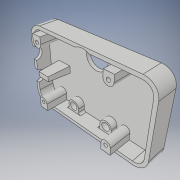
# Autodesk Inventor part: Case_Bottom
Saved by Autodesk Inventor 2019 (Build 230136000, 136)
## iProperties
Created: 2025-01-19
Part Number: Case_Bottom
Material: Générique
Document SubType Name: Modeling
Designer: Maxime
Density: 1 g/cm^3
Appearance: Par défaut
Author: Maxime
Autodesk Inventor part; units mm, degrees
ref_plane "XZ Plane" through (0, 0, 0) normal (0, 1, 0) x (-1, 0, 0)
ref_plane "XY Plane" through (0, 0, 0) normal (0, 0, 1) x (1, 0, 0)
sketch "Esquisse1" plane through (0, 0, 0) normal (0, 0, 1) x (1, 0, 0)
  line L0 (53.2, -33.2) -> (-53.2, -33.2)
  line L1 (-53.2, -33.2) -> (-53.2, 33.2)
  line L2 (-53.2, 33.2) -> (53.2, 33.2)
  line L3 (53.2, 33.2) -> (53.2, -33.2)
  line L4 (53.2, -33.2) -> (-53.2, 33.2) construction
  line L5 (-53.2, -33.2) -> (53.2, 33.2) construction
  point P0 (0, 0)
  dimension "d0" = 66.4
  dimension "d1" = 106.4
  constraints: 12 end point, 2 midpoint, 2 parallel, 1 horizontal, 1 perpendicular
  measures "d0" distance of L0.end L1.end
  measures "d1" distance between parallel lines of L3 L1
extrude "Extrusion1" add sketch "Esquisse1" along normal blind 15.95
shell "Coque1" thickness 3 removed faces 1 at (17.7333, 11.0667, 15.95)
ref_plane "PCBRestingPlane" through (-50.2, -30.2, 22.3) normal (0, 0, 1) x (1, 0, 0)
sketch "Esquisse2" plane through (-50.2, -30.2, 22.3) normal (0, 0, 1) x (1, 0, 0)
  line L0 (75.5, 6.2) -> (12.5, 6.2)
  line L1 (12.5, 6.2) -> (12.5, 55.2)
  line L2 (12.5, 55.2) -> (75.5, 55.2)
  line L3 (75.5, 55.2) -> (75.5, 6.2)
  line L4 (75.5, 6.2) -> (12.5, 55.2) construction
  line L5 (12.5, 6.2) -> (75.5, 55.2) construction
  line L6 (0, 0) -> (0, 60.4) projected
  circle A0 centre (12.5, 55.2) radius 4
  line L7 (8.5, 55.2) -> (8.5, 60.4)
  line L8 (0, 60.4) -> (100.4, 60.4) projected
  line L9 (16.5, 55.2) -> (16.5, 60.4)
  line L10 (16.5, 60.4) -> (8.5, 60.4)
  line L11 (50.2, 30.2) -> (44, 30.7)
  circle A1 centre (12.5, 6.2) radius 4
  line L12 (8.5, 6.2) -> (8.5, 0)
  line L13 (100.4, 0) -> (0, 0) projected
  line L14 (16.5, 6.2) -> (16.5, 0)
  line L15 (8.5, 0) -> (16.5, 0)
  dimension "d6" = 63
  dimension "d7" = 49
  dimension "d8" = 12.5
  dimension "d9" = 8
  dimension "d27" = 8
  dimension "d51" = 0.5
  constraints: 26 end point, 6 point on line, 4 parallel, 4 point on circle, 4 tangent, 3 horizontal, 2 centre point, 2 coincident, 2 midpoint, 2 vertical, 1 perpendicular
  measures "d6" distance of L1.end L2.end
  measures "d7" distance of L0.end L1.end
  measures "d8" distance between parallel lines of L6 L1
  measures "d9" diameter of A0
  measures "d27" diameter of A1
  measures "d51" vertical distance of L11.start L11.end
ref_plane "PCBMiddle" through (-6.2, 0.5, 22.3) normal (1, 0, 0) x (0, 1, 0)
extrude "Extrusion2" add sketch "Esquisse2" against normal up to next contours A1 L1 L0 | L14 L13 L12 A1 | L0 L1 A1 | A0 L1 L2 | L2 L1 A0 | A0 L7 L8 L9
mirror "Symétrie1" about plane through (-6.2, 0.5, 22.3) normal (1, 0, 0) of "Extrusion2"
hole "Perçage2" at (-37.7, 25, 22.3) at (25.3, 25, 22.3) at (25.3, -24, 22.3) at (-37.7, -24, 22.3) direction (0, 0, -1) diameter 3.25 depth 8 start extended yes
sketch "Esquisse4" plane through (-53.2, -33.2, 0) normal (-1, 0, 0) x (0, 0, 1)
  line L0 (15.95, 3) -> (15.95, 63.4) projected
  circle A0 centre (15.95, 42.725) radius 5.6
  circle A1 centre (15.95, 23.675) radius 5.6
  line L1 (15.95, 42.725) -> (15.95, 23.675)
  line L2 (15.95, 66.4) -> (15.95, 0) projected
  line L3 (15.95, 33.2) -> (0, 33.2)
  dimension "d20" = 11.2
  dimension "d21" = 11.2
  dimension "d22" = 19.05
  dimension "d50" = 0
  constraints: 4 end point, 2 centre point, 2 midpoint, 2 point on line, 1 collinear
  measures "d20" diameter of A0
  measures "d21" diameter of A1
  measures "d22" distance of L1.end L1.start
  measures "d50" vertical distance of L3.start L3.end
extrude "Extrusion3" cut sketch "Esquisse4" against normal up to surface (3 mm away)
fillet "Congé2" radius 8 4 edges at (-50.2, 30.2, 9.475) (-50.2, -30.2, 9.475) (50.2, -30.2, 9.475) (50.2, 30.2, 9.475)
fillet "Congé2" radius 11 4 edges at (-53.2, 33.2, 7.975) (-53.2, -33.2, 7.975) (53.2, 33.2, 7.975) (53.2, -33.2, 7.975)
sketch "Esquisse7" plane through (0, 0, 0) normal (0, 0, -1) x (-1, 0, 0)
  circle A0 centre (19, -25) radius 2.5
  circle A1 centre (-13, -25) radius 2.5
  line L0 (-21.3, -30.2) -> (33.7, -30.2) projected
  line L1 (19, -25) -> (-13, -25)
  line L2 (50.2, -22.2) -> (50.2, 22.2) projected
  point P0 (0, 0)
  dimension "d52" = 5
  dimension "d53" = 5
  dimension "d54" = 32
  dimension "d55" = 5.2
  dimension "d58" = 31.2
  constraints: 2 centre point, 2 end point, 1 horizontal
  measures "d52" diameter of A0
  measures "d53" diameter of A1
  measures "d54" distance of L1.start L1.end
  measures "d55" distance from line of L0 L1.start
  measures "d58" distance from line of L2 L1.start
extrude "Extrusion6" cut sketch "Esquisse7" against normal through all
sketch "Esquisse8" plane through (-37.7, 25, 3) normal (0, 0, 1) x (1, 0, 0)
  circle A0 centre (18.7, -50) radius 2.5 projected
  circle A1 centre (18.7, -50) radius 2.5
  line L0 (59, -55.2) -> (4, -55.2) projected
  line L1 (23.9, -44.8) -> (13.5, -44.8)
  line L2 (13.5, -44.8) -> (13.5, -55.2)
  line L3 (13.5, -55.2) -> (23.9, -55.2)
  line L4 (23.9, -55.2) -> (23.9, -44.8)
  line L5 (23.9, -44.8) -> (13.5, -55.2) construction
  line L6 (13.5, -44.8) -> (23.9, -55.2) construction
  point P0 (37.7, -25)
  dimension "d59" = 5
  dimension "d60" = 10.4
  constraints: 12 end point, 2 midpoint, 2 parallel, 1 centre point, 1 coincident, 1 horizontal, 1 perpendicular, 1 point on line
  measures "d59" diameter of A1
  measures "d60" distance of L3.end L2.end
extrude "Extrusion7" add sketch "Esquisse8" along normal blind 6 contours A0 | L0 L2 L1 L4
extrude "Extrusion8" cut sketch "Esquisse8" along normal blind 6 draft 10 contours A0
pattern_linear "Réseau rectangulaire1" count 2 spacing 32 along (1, 0, 0) of "Extrusion8", "Extrusion7"
fillet "Congé3" radius 5.2 4 edges at (-13.8, -19.8, 6) (-24.2, -19.8, 6) (7.8, -19.8, 6) (18.2, -19.8, 6)
fillet "Congé3" radius 2 4 edges at (7.8, -30.2, 6) (-13.8, -30.2, 6) (-24.2, -30.2, 6) (18.2, -30.2, 6)
sketch "Esquisse9" plane through (-37.7, 25, 22.3) normal (0, 0, 1) x (1, 0, 0)
  line L0 (-1.5, -27) -> (8.5, -27)
  line L1 (8.5, -27) -> (8.5, -23)
  line L2 (8.5, -23) -> (-1.5, -23)
  line L3 (-1.5, -23) -> (-1.5, -27)
  line L4 (-1.5, -25) -> (-12.5, -25)
  line L5 (-12.5, -28.925) -> (-12.5, -21.075) projected
  point P0 (37.7, -25)
  dimension "d76" = 4
  dimension "d77" = 10
  dimension "d80" = 11
  constraints: 10 end point, 2 horizontal, 2 midpoint, 2 parallel, 1 perpendicular
  measures "d76" distance of L0.end L1.end
  measures "d77" distance of L0.start L0.end
  measures "d80" distance between parallel lines of L5 L3
extrude "Extrusion9" add sketch "Esquisse9" against normal up to surface (19.3 mm away) draft 3
sketch "Esquisse10" plane through (0, 0, 0) normal (0, 0, -1) x (-1, 0, 0)
  circle A0 centre (1.65, 19.95) radius 9
  line L0 (50.2, -22.2) -> (50.2, 22.2) projected
  line L1 (33.7, 30.2) -> (-21.3, 30.2) projected
  point P0 (0, 0)
  dimension "d81" = 18
  dimension "d82" = 48.55
  dimension "d83" = 10.25
  constraints: 1 centre point
  measures "d81" diameter of A0
  measures "d82" distance from line of L0 A0.centre
  measures "d83" distance from line of L1 A0.centre
extrude "Extrusion10" cut sketch "Esquisse10" against normal through all draft 10
equation "\"d27\" = d9"
equation "\"d21\" = d20"
equation "\"d53\" = d52"
